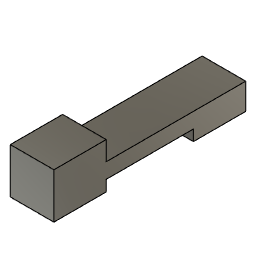
Holder for LED (Autodesk Fusion 360 design; units mm, degrees)
Autodesk Fusion 360 part; units mm, degrees
sketch "Skizze1" plane through (0, 0, 0) normal (0, 0, 1) x (1, 0, 0)
  line L0 (2.5, 11) -> (-2.5, 11)
  line L1 (-2.5, 11) -> (-2.5, -11)
  line L2 (-2.5, -11) -> (2.5, -11)
  line L3 (2.5, -11) -> (2.5, 11)
  line L4 (2.5, 11) -> (-2.5, -11) construction
  line L5 (-2.5, 11) -> (2.5, -11) construction
  line L6 (-2.5, -11) -> (2.5, -11)
  line L7 (2.5, -11) -> (2.5, -5)
  line L8 (2.5, -5) -> (-2.5, -5)
  line L9 (-2.5, -5) -> (-2.5, -11)
  line L10 (2.5, -5) -> (2.5, 5) construction
  line L11 (2.5, 5) -> (-2.5, 5)
  dimension "d1" = 5
  dimension "d2" = 22
  dimension "d3" = 5
  dimension "d4" = 6
  dimension "d13" = 10
  constraint perpendicular L0 L1
  constraint parallel L0 L2
  constraint parallel L1 L3
  constraint horizontal L0
  constraint coincident L4 origin
  constraint coincident L5 origin
  constraint horizontal L6
  constraint vertical L7
  constraint horizontal L8
  constraint vertical L9
  constraint perpendicular L8 L10
  constraint coincident L1 L11.end
  constraint perpendicular L1 L11
  measures "d1" distance of L1.end L2.end L0.end
  measures "d2" distance of L0.end L1.end
  measures "d3" distance of L1.end L2.end
  measures "d4" distance of L1.end L8.end
  measures "d13" distance of L7.end L10.end
extrude "Extrusion4" add sketch "Skizze1" along normal blind 3
extrude "Extrusion5" add sketch "Skizze1" along normal blind 5.2 contours L1 L2 L3 L6 L7 L8 L9
extrude "Extrusion6" cut sketch "Skizze1" along normal blind 1.25 contours L1 L3 L8 L11
named bodies: "Holder"
